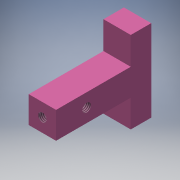
# Autodesk Inventor part: vexSupportForArm
Saved by Autodesk Inventor 2016 SP1 (Build 200210100, 210)
## iProperties
Created: 2015-07-13
Part Number: vexSupportForArm
Material: Aluminum 6061
Document SubType Name: Modeling
Designer: steele
Density: 2.7 g/cm^3
Appearance: Pink
Mass: 94.7579 g
Surface Area: 105.47 cm^2
Volume: 35.0955 cm^3
Author: steele
Autodesk Inventor part; units mm, degrees
ref_plane "YZ Plane" through (0, 0, 0) normal (1, 0, 0) x (0, 1, 0)
ref_plane "XZ Plane" through (0, 0, 0) normal (0, 1, 0) x (-1, 0, 0)
ref_plane "XY Plane" through (0, 0, 0) normal (0, 0, 1) x (1, 0, 0)
sketch "Sketch1" plane through (0, 0, 0) normal (0, 0, 1) x (1, 0, 0)
  line L0 (-6.35, -19.05) -> (6.35, -19.05)
  line L1 (6.35, -19.05) -> (6.35, 19.05)
  line L2 (6.35, 19.05) -> (-6.35, 19.05)
  line L3 (-6.35, 19.05) -> (-6.35, -19.05)
  line L4 (-6.35, -19.05) -> (6.35, 19.05) construction
  line L5 (6.35, -19.05) -> (-6.35, 19.05) construction
  point P0 (0, 0)
  dimension "height" = 38.1
  dimension "width" = 12.7
  constraints: 12 end point, 2 midpoint, 2 parallel, 1 horizontal, 1 perpendicular
  measures "height" distance of L0.end L1.end
  measures "width" distance of L1.end L2.end
extrude "Extrusion9" add sketch "Sketch1" against normal blind 9.525
sketch "Sketch19" plane through (0, 0, 0) normal (0, 0, 1) x (1, 0, 0)
  line L0 (-6.35, -6.223) -> (6.35, -6.223)
  line L1 (6.35, -6.223) -> (6.35, 6.223)
  line L2 (6.35, 6.223) -> (-6.35, 6.223)
  line L3 (-6.35, 6.223) -> (-6.35, -6.223)
  line L4 (-6.35, -6.223) -> (6.35, 6.223) construction
  line L5 (6.35, -6.223) -> (-6.35, 6.223) construction
  line L6 (-6.35, 19.05) -> (-6.35, -19.05) projected
  point P0 (0, 0)
  dimension "d126" = 12.446
  constraints: 12 end point, 2 midpoint, 2 parallel, 1 collinear, 1 perpendicular
  measures "d126" distance of L2.end L0.start
extrude "Extrusion10" add sketch "Sketch19" along normal blind 34.798
sketch "Sketch20" plane through (6.35, -19.05, -9.525) normal (1, 0, 0) x (0, 0, -1)
  line L0 (-9.525, 25.273) -> (-9.525, 38.1) projected
  line L1 (-9.525, 19.05) -> (-44.323, 19.05) construction
  line L2 (-44.323, 25.273) -> (-44.323, 12.827) construction
  point P0 (-30.099, 19.05)
  dimension "d129" = 20.574
  dimension "d137" = 0
  constraints: 2 end point, 1 midpoint
  measures "d129" distance from line of point (-30.099, 19.05) L0
  measures "d137" distance from line of point (-30.099, 19.05) L1
hole "Hole13" at (6.35, 0, 20.574) direction (-1, 0, 0) diameter 3.9624 end through all thread size "10-32 UNF" class "2B" standard "ANSI Unified Screw Threads"
sketch "Sketch21" plane through (0, 0, 34.798) normal (0, 0, 1) x (1, 0, 0)
  point P0 (0, 0)
  point P1 (0, 0)
  constraints: 1 coincident
hole "Hole14" at (0, 0, 34.798) direction (0, 0, -1) diameter 3.9624 depth 10.16 tip angle 118 thread size "10-32 UNF" class "2B" standard "ANSI Unified Screw Threads"
sketch "Sketch22" plane through (-6.35, -6.223, 0) normal (0, -1, 0) x (1, 0, 0)
  point P0 (6.35, 0)
sketch "Sketch23" plane through (-6.35, -6.223, 0) normal (0, -1, 0) x (1, 0, 0)
  line L0 (0, 34.798) -> (12.7, 34.798) projected
  point P0 (6.35, 0)
  point P1 (6.35, 9.398)
  dimension "d145" = 25.4
  measures "d145" distance from line of point (6.35, 9.398) L0
hole "Hole15" at (0, -6.223, 9.398) direction (0, 1, 0) diameter 3.9624 end through all thread size "10-32 UNF" class "2B" standard "ANSI Unified Screw Threads"
equation "\"height\" = partHeight"
equation "\"width\" = partWidth"
equation "\"d124\" = depthBehindPlate"
equation "\"d126\" = slotWidth"
equation "\"d127\" = 2 * centerLineOfCylinder + plateThickness"
equation "\"d129\" = centerLineOfCylinder + plateThickness"
equation "\"partWidth\" = 12.7"
equation "\"centerLineOfCylinder\" = 14.224"
equation "\"partHeight\" = 38.1"
equation "\"depthBehindPlate\" = 9.525"
equation "\"plateThickness\" = 6.35"
equation "\"printerOffset\" = 0.254"
equation "\"slotWidth\" = 12.446"
body "Solid2"
